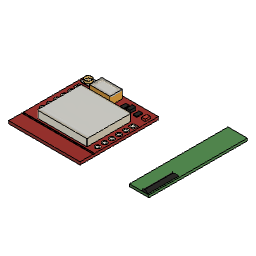
Sim800L Board + Antenna (Autodesk Fusion 360 design; units mm, degrees)
Autodesk Fusion 360 part; units mm, degrees
note: some values were not read from the file. Set by a fixed rule: which sketch regions a step uses.
sketch "Sketch1" plane through (0, 0, 0) normal (0, 0, 1) x (1, 0, 0)
  line L0 (12.75, 14) -> (-12.75, 14)
  line L1 (-12.75, 14) -> (-12.75, -14)
  line L2 (-12.75, -14) -> (12.75, -14)
  line L3 (12.75, -14) -> (12.75, 14)
  line L4 (12.75, 14) -> (-12.75, -14) construction
  line L5 (-12.75, 14) -> (12.75, -14) construction
  dimension "d1" = 25.5
  dimension "d2" = 28
  constraint horizontal L0
  constraint perpendicular L0 L1
  constraint parallel L0 L2
  constraint parallel L1 L3
  constraint coincident L4 origin
  constraint coincident L5 origin
  measures "d1" distance of L1.end L2.end
  measures "d2" distance of L0.end L1.end
extrude "Extrude1" add sketch "Sketch1" along normal blind 1 makes body 1
sketch "Sketch2" plane through (0, 0, 1) normal (0, 0, 1) x (-1, 0, 0)
  line L0 (-12.75, 14) -> (-12.75, -14)
  line L1 (-12.75, -14) -> (12.75, -14)
  line L2 (12.75, -14) -> (12.75, 14)
  line L3 (12.75, 14) -> (-12.75, 14)
  line L4 (12.75, 8.75) -> (-12.75, 8.75)
  line L5 (-12.75, 8.75) -> (-12.75, 9.25)
  line L6 (-12.75, 9.25) -> (12.75, 9.25)
  line L7 (12.75, 9.25) -> (12.75, 8.75)
  dimension "d5" = 0.5
  dimension "d6" = 4.75
  constraint horizontal L4
  constraint vertical L5
  constraint horizontal L6
  constraint vertical L7
  constraint coincident L0 L5.end
  constraint coincident L2 L4.start
  measures "d5" distance of L4.end L5.end
  measures "d6" distance of L3 L6
extrude "Extrude2" cut sketch "Sketch2" against normal blind 0.15 contours L0 L2 L4 L5 L6 L7 bodies 1
sketch "Sketch3" plane through (0, 0, 1) normal (0, 0, 1) x (-1, 0, 0)
  line L0 (12.75, 8.75) -> (-12.75, 8.75)
  line L1 (-12.75, 8.75) -> (-12.75, -14)
  line L2 (-12.75, -14) -> (12.75, -14)
  line L3 (12.75, -14) -> (12.75, 8.75)
  line L4 (8.45, -7.7) -> (-9.35, -7.7)
  line L5 (-9.35, -7.7) -> (-9.35, 8.1)
  line L6 (-9.35, 8.1) -> (8.45, 8.1)
  line L7 (8.45, 8.1) -> (8.45, -7.7)
  dimension "d9" = 17.8
  dimension "d10" = 15.8
  dimension "d11" = 3.4
  dimension "d12" = 6.8
  dimension "d13" = 6.3
  constraint horizontal L4
  constraint vertical L5
  constraint horizontal L6
  constraint vertical L7
  measures "d9" distance of L4.start L4.end
  measures "d10" distance of L4.end L5.end
  measures "d11" distance of L1 L5
  measures "d13" distance of L2 L4
extrude "Extrude3" add sketch "Sketch3" along normal blind 2.5 contours L4 L5 L6 L7 bodies 1
sketch "Sketch4" plane through (0, 0, 1) normal (0, 0, 1) x (-1, 0, 0)
  line L0 (8.45, 8.1) -> (8.45, -7.7)
  line L1 (8.45, -7.7) -> (-9.35, -7.7)
  line L2 (-9.35, -7.7) -> (-9.35, 8.1)
  line L3 (-9.35, 8.1) -> (8.45, 8.1)
  line L4 (12.75, 8.75) -> (-12.75, 8.75)
  line L5 (-12.75, 8.75) -> (-12.75, -14)
  line L6 (-12.75, -14) -> (12.75, -14)
  line L7 (12.75, -14) -> (12.75, 8.75)
  line L8 (6.45, -13) -> (-0.85, -13)
  line L9 (-0.85, -13) -> (-0.85, -8.6)
  line L10 (-0.85, -8.6) -> (6.45, -8.6)
  line L11 (6.45, -8.6) -> (6.45, -13)
  dimension "d16" = 4.4
  dimension "d17" = 7.3
  dimension "d18" = 1
  dimension "d19" = 6.3
  constraint horizontal L8
  constraint vertical L9
  constraint horizontal L10
  constraint vertical L11
  measures "d16" distance of L8.end L9.end
  measures "d17" distance of L8.start L8.end
  measures "d18" distance of L6 L8
  measures "d19" distance of L7 L11
extrude "Extrude4" add sketch "Sketch4" along normal blind 3 contours L8 L9 L10 L11 bodies 1
sketch "Sketch5" plane through (0, 0, 1) normal (0, 0, 1) x (-1, 0, 0)
  line L0 (6.45, -8.6) -> (6.45, -13)
  line L1 (6.45, -13) -> (-0.85, -13)
  line L2 (-0.85, -13) -> (-0.85, -8.6)
  line L3 (-0.85, -8.6) -> (6.45, -8.6)
  line L4 (8.45, 8.1) -> (8.45, -7.7)
  line L5 (8.45, -7.7) -> (-9.35, -7.7)
  line L6 (-9.35, -7.7) -> (-9.35, 8.1)
  line L7 (-9.35, 8.1) -> (8.45, 8.1)
  line L8 (12.75, 8.75) -> (-12.75, 8.75)
  line L9 (-12.75, 8.75) -> (-12.75, -14)
  line L10 (-12.75, -14) -> (12.75, -14)
  line L11 (12.75, -14) -> (12.75, 8.75)
  line L12 (-3.05, -12) -> (-4.35, -12)
  line L13 (-4.35, -12) -> (-4.35, -10)
  line L14 (-4.35, -10) -> (-3.05, -10)
  line L15 (-3.05, -10) -> (-3.05, -12)
  line L16 (-5.45, -12) -> (-6.75, -12)
  line L17 (-6.75, -12) -> (-6.75, -9.9)
  line L18 (-6.75, -9.9) -> (-5.45, -9.9)
  line L19 (-5.45, -9.9) -> (-5.45, -12)
  line L20 (-7.85, -12) -> (-9.15, -12)
  line L21 (-9.15, -12) -> (-9.15, -9.9)
  line L22 (-9.15, -9.9) -> (-7.85, -9.9)
  line L23 (-7.85, -9.9) -> (-7.85, -12)
  line L24 (-10.65, -11.9) -> (-11.95, -11.9)
  line L25 (-11.95, -11.9) -> (-11.95, -10.1)
  line L26 (-11.95, -10.1) -> (-10.65, -10.1)
  line L27 (-10.65, -10.1) -> (-10.65, -11.9)
  dimension "d22" = 2
  dimension "d23" = 1.3
  dimension "d24" = 2
  dimension "d25" = 9.7
  dimension "d26" = 1.3
  dimension "d27" = 2.1
  dimension "d28" = 7.3
  dimension "d29" = 2
  dimension "d30" = 2.1
  dimension "d31" = 1.3
  dimension "d32" = 2
  dimension "d33" = 4.9
  dimension "d34" = 1.3
  dimension "d35" = 1.8
  dimension "d36" = 2.1
  dimension "d37" = 2.1
  constraint horizontal L12
  constraint vertical L13
  constraint horizontal L14
  constraint vertical L15
  constraint horizontal L16
  constraint vertical L17
  constraint horizontal L18
  constraint vertical L19
  constraint horizontal L20
  constraint vertical L21
  constraint horizontal L22
  constraint vertical L23
  constraint horizontal L24
  constraint vertical L25
  constraint horizontal L26
  constraint vertical L27
  measures "d22" distance of L12.end L13.end
  measures "d23" distance of L12.start L12.end
  measures "d24" distance of L10 L12
  measures "d25" distance of L9 L15
  measures "d26" distance of L16.start L16.end
  measures "d27" distance of L16.end L17.end
  measures "d28" distance of L9 L19
  measures "d29" distance of L10 L16
  measures "d30" distance of L20.end L21.end
  measures "d31" distance of L20.start L20.end
  measures "d32" distance of L10 L20
  measures "d33" distance of L9 L23
  measures "d34" distance of L24.start L24.end
  measures "d35" distance of L24.end L25.end
  measures "d36" distance of L10 L24
  measures "d37" distance of L9 L27
extrude "Extrude5" add sketch "Sketch5" along normal blind 0.3 contours L12 L13 L14 L15 bodies 1
extrude "Extrude6" add sketch "Sketch5" along normal blind 1 contours L16 L17 L18 L19 bodies 1
extrude "Extrude7" add sketch "Sketch5" along normal blind 0.3 contours L20 L21 L22 L23 bodies 1
extrude "Extrude8" add sketch "Sketch5" along normal blind 0.75 contours L24 L25 L26 L27 bodies 1
sketch "Sketch6" plane through (0, 0, 1) normal (0, 0, 1) x (-1, 0, 0)
  circle A0 centre (10.58, -12.3) radius 1.25
  circle A1 centre (10.58, -12.3) radius 1.15
  circle A2 centre (10.58, -12.3) radius 0.25
  line L0 (12.08, -10.8) -> (9.08, -10.8)
  line L1 (9.08, -10.8) -> (9.08, -13.8)
  line L2 (9.08, -13.8) -> (12.08, -13.8)
  line L3 (12.08, -13.8) -> (12.08, -10.8)
  line L4 (12.08, -10.8) -> (9.08, -13.8) construction
  line L5 (9.08, -10.8) -> (12.08, -13.8) construction
  line L6 (-12.75, -14) -> (12.75, -14)
  line L7 (12.75, -14) -> (12.75, 8.75)
  point P0 (10.58, -12.3)
  dimension "d46" = 2.5
  dimension "d47" = 0.1
  dimension "d48" = 0.5
  dimension "d49" = 3
  dimension "d50" = 3
  dimension "d51" = 0.2
  dimension "d52" = 0.67
  constraint concentric A0 A1
  constraint concentric A0 A2
  constraint horizontal L0
  constraint perpendicular L0 L1
  constraint parallel L0 L2
  constraint parallel L1 L3
  constraint coincident L4 P0
  constraint coincident L5 P0
  constraint coincident P0 A0.centre
  measures "d46" diameter of A0
  measures "d47" distance of A0 A1
  measures "d48" diameter of A2
  measures "d49" distance of L0.start L0.end
  measures "d50" distance of L0.start L2.end
  measures "d51" distance of L2 L6
  measures "d52" distance of L3 L7
extrude "Extrude9" add sketch "Sketch6" along normal blind 1 contours A0 | A2 bodies 1
extrude "Extrude10" add sketch "Sketch6" along normal blind 0.2 bodies 1
sketch "Sketch7" plane through (0, 0, 1) normal (0, 0, 1) x (-1, 0, 0)
  line L0 (12.08, -13.8) -> (9.08, -13.8)
  line L1 (9.08, -13.8) -> (9.08, -10.8)
  line L2 (9.08, -10.8) -> (12.08, -10.8)
  line L3 (12.08, -10.8) -> (12.08, -13.8)
  line L4 (12.75, 8.75) -> (-12.75, 8.75)
  line L5 (-12.75, 8.75) -> (-12.75, -14)
  line L6 (-12.75, -14) -> (12.75, -14)
  line L7 (12.75, -14) -> (12.75, 8.75)
  line L8 (8.45, 8.1) -> (8.45, -7.7)
  line L9 (8.45, -7.7) -> (-9.35, -7.7)
  line L10 (-9.35, -7.7) -> (-9.35, 8.1)
  line L11 (-9.35, 8.1) -> (8.45, 8.1)
  line L12 (6.45, -8.6) -> (6.45, -13)
  line L13 (6.45, -13) -> (-0.85, -13)
  line L14 (-0.85, -13) -> (-0.85, -8.6)
  line L15 (-0.85, -8.6) -> (6.45, -8.6)
  line L16 (-3.05, -10) -> (-3.05, -12)
  line L17 (-3.05, -12) -> (-4.35, -12)
  line L18 (-4.35, -12) -> (-4.35, -10)
  line L19 (-4.35, -10) -> (-3.05, -10)
  line L20 (-5.45, -9.9) -> (-5.45, -12)
  line L21 (-5.45, -12) -> (-6.75, -12)
  line L22 (-6.75, -12) -> (-6.75, -9.9)
  line L23 (-6.75, -9.9) -> (-5.45, -9.9)
  line L24 (-7.85, -9.9) -> (-7.85, -12)
  line L25 (-7.85, -12) -> (-9.15, -12)
  line L26 (-9.15, -12) -> (-9.15, -9.9)
  line L27 (-9.15, -9.9) -> (-7.85, -9.9)
  line L28 (-10.65, -10.1) -> (-10.65, -11.9)
  line L29 (-10.65, -11.9) -> (-11.95, -11.9)
  line L30 (-11.95, -11.9) -> (-11.95, -10.1)
  line L31 (-11.95, -10.1) -> (-10.65, -10.1)
  line L32 (-11.25, 8.75) -> (-11.25, -14) construction
  line L33 (10.75, 8.75) -> (10.75, -14) construction
  circle A0 centre (-11.25, -6.5) radius 0.6
  circle A1 centre (-11.25, -3.96) radius 0.6
  circle A2 centre (-11.25, -1.42) radius 0.6
  circle A3 centre (-11.25, 1.12) radius 0.6
  circle A4 centre (-11.25, 3.66) radius 0.6
  circle A5 centre (-11.25, 6.2) radius 0.6
  circle A6 centre (10.75, -9) radius 0.6
  circle A7 centre (10.75, -6.46) radius 0.6
  circle A8 centre (10.75, -3.92) radius 0.6
  circle A9 centre (10.75, -1.38) radius 0.6
  circle A10 centre (10.75, 1.16) radius 0.6
  circle A11 centre (10.75, 3.7) radius 0.6
  dimension "d57" = 1.5
  dimension "d58" = 2
  dimension "d59" = 7.5
  dimension "d60" = 1.2
  dimension "d63" = -2.54
  dimension "d64" = 0
  dimension "d65" = 1.2
  dimension "d66" = 5
  dimension "d69" = 0
  dimension "d70" = 2.54
  constraint coincident L4 L32.start
  constraint coincident L6 L32.end
  constraint perpendicular L6 L32
  constraint coincident L4 L33.start
  constraint coincident L6 L33.end
  constraint perpendicular L6 L33
  constraint coincident L32 A0.centre
  constraint coincident L33 A6.centre
  measures "d57" distance of L5 L32
  measures "d58" distance of L7 L33
  measures "d59" distance of L32.end A0.centre
  measures "d60" diameter of A0
  measures "d65" diameter of A6
  measures "d66" distance of L6 A6.centre
extrude "Extrude11" cut sketch "Sketch7" against normal up to surface (1 mm away) contours A0 | A1 | A2 | A3 | A4 | A5 | A6 | A7 | A8 | A9 | A10 | A11 bodies 1
sketch "Sketch8" plane through (0, 0, 0) normal (0, 0, -1) x (1, 0, 0)
  circle A0 centre (11.25, -1.42) radius 0.6
  circle A1 centre (-10.75, 3.7) radius 0.6
  circle A2 centre (-10.75, -6.46) radius 0.6
  circle A3 centre (-10.75, -3.92) radius 0.6
  circle A4 centre (11.25, 6.2) radius 0.6
  circle A5 centre (11.25, -3.96) radius 0.6
  circle A6 centre (11.25, 1.12) radius 0.6
  circle A7 centre (-10.75, 1.16) radius 0.6
  circle A8 centre (-10.75, -9) radius 0.6
  circle A9 centre (-10.75, -1.38) radius 0.6
  circle A10 centre (11.25, 3.66) radius 0.6
  circle A11 centre (11.25, -6.5) radius 0.6
  line L0 (12.75, -14) -> (12.75, 14)
  line L1 (12.75, 14) -> (-12.75, 14)
  line L2 (-12.75, 14) -> (-12.75, -14)
  line L3 (-12.75, -14) -> (12.75, -14)
  line L4 (-7.35, -13.95) -> (8.05, -13.95)
  line L5 (8.05, -13.95) -> (8.05, 3.25)
  line L6 (8.05, 3.25) -> (3.25, 3.25)
  line L7 (3.25, 3.25) -> (3.25, 1.95)
  line L8 (3.25, 1.95) -> (-7.35, 1.95)
  line L9 (-7.35, 1.95) -> (-7.35, -13.95)
  dimension "d73" = 15.4
  dimension "d75" = 10.6
  dimension "d76" = 1.3
  dimension "d77" = 15.9
  dimension "d108" = 0.05
  dimension "d109" = 20.1
  constraint perpendicular L5 L6
  constraint perpendicular L6 L7
  constraint perpendicular L5 L8
  constraint horizontal L8
  constraint vertical L9
  measures "d73" distance of L4.start L4.end
  measures "d75" distance of L7.end L8.end
  measures "d76" distance of L6 L8
  measures "d77" distance of L4.start L8.end
  measures "d108" distance of L3 L4
  measures "d109" distance of L0.start L9
extrude "Extrude12" add sketch "Sketch8" along normal blind 1.3 contours L4 L5 L6 L7 L8 L9 bodies 1
ref_plane "WorkPlane1" through (0, 0, -0.4) normal (0, 0, -1) x (-1, 0, 0)
sketch "Sketch10" plane through (0, 0, -0.4) normal (0, 0, -1) x (1, 0, 0)
  line L0 (-6.85, -0.3) -> (5.15, -0.3)
  line L1 (5.15, -0.3) -> (5.15, -15.1)
  line L2 (5.15, -15.1) -> (-6.85, -15.1)
  line L3 (-6.85, -15.1) -> (-6.85, -0.3)
  line L4 (12.75, -14) -> (-12.75, -14)
  line L5 (-7.35, 1.95) -> (-7.35, -13.95)
  point P0 (-7.35, -13.95)
  dimension "d90" = 12
  dimension "d91" = 14.8
  dimension "d110" = 1.1
  dimension "d111" = 0.5
  constraint horizontal L0
  constraint vertical L1
  constraint horizontal L2
  constraint vertical L3
  measures "d90" distance of L0.start L0.end
  measures "d91" distance of L0.start L2.end
  measures "d110" distance of L1.end L4
  measures "d111" distance of L2.end L5
extrude "Extrude14" cut sketch "Sketch10" along normal blind 0.75 bodies 1
sketch "Sketch9" plane through (0, 0, -0.4) normal (0, 0, -1) x (1, 0, 0)
  line L0 (5.15, -0.25) -> (5.15, -12.25)
  line L1 (5.15, -12.25) -> (2.35, -15.05)
  line L2 (2.35, -15.05) -> (-6.85, -15.05)
  line L3 (-6.85, -15.05) -> (-6.85, -0.25)
  line L4 (-6.85, -0.25) -> (5.15, -0.25)
  line L5 (8.05, -13.95) -> (-7.35, -13.95)
  dimension "d82" = 12
  dimension "d83" = 9.2
  dimension "d84" = 45
  dimension "d96" = 14.8
  dimension "d112" = 1.1
  dimension "d113" = 0.5
  constraint perpendicular L0 L2
  constraint perpendicular L2 L3
  constraint perpendicular L0 L4
  measures "d82" distance of L0 L3
  measures "d83" distance of L1.end L2.end
  measures "d84" angle of L0 L1
  measures "d96" distance of L2.end L3.end
  measures "d112" distance of L2 L5
  measures "d113" distance of L3 L5.end
extrude "Extrude13" add sketch "Sketch9" along normal blind 0.7 separate body makes body 2
fillet "Fillet1" radius 0.5 5 edges at (2.35, 15.05, -0.75) (-6.85, 15.05, -0.75) (5.15, 12.25, -0.75) (5.15, 0.25, -0.75) (-6.85, 0.25, -0.75) on bodies 2
sketch "Sketch11" plane through (0, 0, 1) normal (0, 0, 1) x (-1, 0, 0)
  circle A0 centre (-11.25, -1.42) radius 0.6
  circle A1 centre (10.75, 3.7) radius 0.6
  circle A2 centre (10.75, -6.46) radius 0.6
  circle A3 centre (10.75, -3.92) radius 0.6
  circle A4 centre (-11.25, 6.2) radius 0.6
  circle A5 centre (-11.25, -3.96) radius 0.6
  circle A6 centre (-11.25, 1.12) radius 0.6
  circle A7 centre (10.75, 1.16) radius 0.6
  circle A8 centre (10.75, -9) radius 0.6
  circle A9 centre (10.75, -1.38) radius 0.6
  circle A10 centre (-11.25, 3.66) radius 0.6
  circle A11 centre (-11.25, -6.5) radius 0.6
  line L0 (12.08, -13.8) -> (9.08, -13.8)
  line L1 (9.08, -13.8) -> (9.08, -10.8)
  line L2 (9.08, -10.8) -> (12.08, -10.8)
  line L3 (12.08, -10.8) -> (12.08, -13.8)
  line L4 (12.75, 8.75) -> (-12.75, 8.75)
  line L5 (-12.75, 8.75) -> (-12.75, -14)
  line L6 (-12.75, -14) -> (12.75, -14)
  line L7 (12.75, -14) -> (12.75, 8.75)
  line L8 (8.45, 8.1) -> (8.45, -7.7)
  line L9 (8.45, -7.7) -> (-9.35, -7.7)
  line L10 (-9.35, -7.7) -> (-9.35, 8.1)
  line L11 (-9.35, 8.1) -> (8.45, 8.1)
  line L12 (6.45, -8.6) -> (6.45, -13)
  line L13 (6.45, -13) -> (-0.85, -13)
  line L14 (-0.85, -13) -> (-0.85, -8.6)
  line L15 (-0.85, -8.6) -> (6.45, -8.6)
  line L16 (-3.05, -10) -> (-3.05, -12)
  line L17 (-3.05, -12) -> (-4.35, -12)
  line L18 (-4.35, -12) -> (-4.35, -10)
  line L19 (-4.35, -10) -> (-3.05, -10)
  line L20 (-5.45, -9.9) -> (-5.45, -12)
  line L21 (-5.45, -12) -> (-6.75, -12)
  line L22 (-6.75, -12) -> (-6.75, -9.9)
  line L23 (-6.75, -9.9) -> (-5.45, -9.9)
  line L24 (-7.85, -9.9) -> (-7.85, -12)
  line L25 (-7.85, -12) -> (-9.15, -12)
  line L26 (-9.15, -12) -> (-9.15, -9.9)
  line L27 (-9.15, -9.9) -> (-7.85, -9.9)
  line L28 (-10.65, -10.1) -> (-10.65, -11.9)
  line L29 (-10.65, -11.9) -> (-11.95, -11.9)
  line L30 (-11.95, -11.9) -> (-11.95, -10.1)
  line L31 (-11.95, -10.1) -> (-10.65, -10.1)
  line L32 (-12.15, -7.4) -> (-10.35, -7.4)
  line L33 (-10.35, -7.4) -> (-10.35, -5.6)
  line L34 (-10.35, -5.6) -> (-12.15, -5.6)
  line L35 (-12.15, -5.6) -> (-12.15, -7.4)
  line L36 (-12.15, -7.4) -> (-10.35, -5.6) construction
  line L37 (-10.35, -7.4) -> (-12.15, -5.6) construction
  line L38 (9.85, -9.9) -> (11.65, -9.9)
  line L39 (11.65, -9.9) -> (11.65, -8.1)
  line L40 (11.65, -8.1) -> (9.85, -8.1)
  line L41 (9.85, -8.1) -> (9.85, -9.9)
  line L42 (9.85, -9.9) -> (11.65, -8.1) construction
  line L43 (11.65, -9.9) -> (9.85, -8.1) construction
  circle A12 centre (10.75, -6.46) radius 0.9
  circle A13 centre (10.75, -3.92) radius 0.9
  circle A14 centre (10.75, -1.38) radius 0.9
  circle A15 centre (10.75, 1.16) radius 0.9
  circle A16 centre (10.75, 3.7) radius 0.9
  circle A17 centre (-11.25, 6.2) radius 0.9
  circle A18 centre (-11.25, 3.66) radius 0.9
  circle A19 centre (-11.25, 1.12) radius 0.9
  circle A20 centre (-11.25, -1.42) radius 0.9
  circle A21 centre (-11.25, -3.96) radius 0.9
  point P0 (-11.25, -6.5)
  point P1 (10.75, -9)
  dimension "d97" = 1.8
  dimension "d98" = 1.8
  dimension "d99" = 1.8
  dimension "d100" = 1.8
  dimension "d103" = 1.8
  dimension "d104" = 1.8
  constraint horizontal L32
  constraint perpendicular L32 L33
  constraint parallel L32 L34
  constraint parallel L33 L35
  constraint coincident L36 P0
  constraint coincident L37 P0
  constraint coincident P0 A11.centre
  constraint horizontal L38
  constraint perpendicular L38 L39
  constraint parallel L38 L40
  constraint parallel L39 L41
  constraint coincident L42 P1
  constraint coincident L43 P1
  constraint coincident P1 A8.centre
  constraint concentric A2 A12
  constraint concentric A3 A13
  constraint concentric A9 A14
  constraint concentric A7 A15
  constraint concentric A1 A16
  constraint concentric A4 A17
  constraint concentric A10 A18
  constraint concentric A6 A19
  constraint concentric A0 A20
  constraint concentric A5 A21
  constraint equal A12 A14
  constraint equal A14 A15
  constraint equal A15 A16
  constraint equal A16 A21
  constraint equal A20 A21
  constraint equal A19 A20
  constraint equal A18 A19
  constraint equal A17 A18
  measures "d97" distance of L33.end L34.end
  measures "d98" distance of L32.end L33.end
  measures "d99" distance of L39.end L40.end
  measures "d100" distance of L38.end L39.end
  measures "d103" diameter of A12
  measures "d104" diameter of A13
extrude "Extrude15" cut sketch "Sketch11" against normal blind 0.01 contours L32 L33 L34 L35 | L38 L39 L40 L41 | A12 | A13 | A14 | A15 | A16 | A17 | A18 | A19 | A20 | A21 bodies 1
fillet "Fillet2" radius 0.2 4 edges at (-12.08, 13.8, 1.1) (-9.08, 13.8, 1.1) (-12.08, 10.8, 1.1) (-9.08, 10.8, 1.1) on bodies 1
fillet "Fillet3" radius 0.3 4 edges at (9.35, -8.1, 2.25) (-8.45, -8.1, 2.25) (9.35, 7.7, 2.25) (-8.45, 7.7, 2.25) on bodies 1
sketch "Sketch12" plane through (0, 0, 0) normal (0, 0, 1) x (1, 0, 0)
  line L0 (28.2729, 23.3773) -> (35.1729, 23.3773)
  line L1 (35.1729, 23.3773) -> (35.1729, -11.8227)
  line L2 (35.1729, -11.8227) -> (28.2729, -11.8227)
  line L3 (28.2729, -11.8227) -> (28.2729, 23.3773)
  dimension "d114" = 35.2
  dimension "d115" = 6.9
  constraint horizontal L0
  constraint vertical L1
  constraint horizontal L2
  constraint vertical L3
  measures "d114" distance of L0.end L1.end
  measures "d115" distance of L0.start L0.end
extrude "Extrude16" add sketch "Sketch12" along normal blind 0.85 separate body makes body 3
sketch "Sketch13" plane through (0, 0, 0.85) normal (0, 0, 1) x (-1, 0, 0)
  line L0 (-28.2729, 11.8227) -> (-35.1729, 11.8227)
  line L1 (-35.1729, 11.8227) -> (-35.1729, -23.3773)
  line L2 (-35.1729, -23.3773) -> (-28.2729, -23.3773)
  line L3 (-28.2729, -23.3773) -> (-28.2729, 11.8227)
  line L4 (-32.6729, 0.8227) -> (-34.6729, 0.8227)
  line L5 (-34.6729, 0.8227) -> (-34.6729, 11.8127)
  line L6 (-34.6729, 11.8127) -> (-32.6729, 11.8127)
  line L7 (-32.6729, 11.8127) -> (-32.6729, 0.8227)
  dimension "d118" = 2
  dimension "d119" = 0.5
  dimension "d120" = 11
  dimension "d124" = 0.01
  constraint horizontal L4
  constraint vertical L5
  constraint horizontal L6
  constraint vertical L7
  measures "d118" distance of L4.start L4.end
  measures "d119" distance of L1 L5.end
  measures "d120" distance of L0 L4.end
  measures "d124" distance of L0 L6
extrude "Extrude17" add sketch "Sketch13" along normal blind 1 contours L4 L5 L6 L7 bodies 3
fillet "Fillet4" radius 0.99 3 edges at (32.6729, -6.3177, 1.85) (34.6729, -6.3177, 1.85) (33.6729, -0.8227, 1.85) on bodies 3
sketch "Sketch14" plane through (0, 0, 0) normal (0, 0, -1) x (1, 0, 0)
  line L0 (-7.35, 1.95) -> (3.25, 1.95)
  line L1 (3.25, 1.95) -> (3.25, 3.25)
  line L2 (3.25, 3.25) -> (8.05, 3.25)
  line L3 (8.05, 3.25) -> (8.05, -13.95)
  line L4 (8.05, -13.95) -> (-7.35, -13.95)
  line L5 (-7.35, -13.95) -> (-7.35, 1.95)
  circle A0 centre (11.25, -1.42) radius 0.6
  circle A1 centre (-10.75, 3.7) radius 0.6
  circle A2 centre (-10.75, -6.46) radius 0.6
  circle A3 centre (-10.75, -3.92) radius 0.6
  circle A4 centre (11.25, 6.2) radius 0.6
  circle A5 centre (11.25, -3.96) radius 0.6
  circle A6 centre (11.25, 1.12) radius 0.6
  circle A7 centre (-10.75, 1.16) radius 0.6
  circle A8 centre (-10.75, -9) radius 0.6
  circle A9 centre (-10.75, -1.38) radius 0.6
  circle A10 centre (11.25, 3.66) radius 0.6
  circle A11 centre (11.25, -6.5) radius 0.6
  line L6 (12.75, -14) -> (12.75, 14)
  line L7 (12.75, 14) -> (-12.75, 14)
  line L8 (-12.75, 14) -> (-12.75, -14)
  line L9 (-12.75, -14) -> (12.75, -14)
  circle A12 centre (-10.75, 3.7) radius 0.9
  circle A13 centre (-10.75, 1.16) radius 0.9
  circle A14 centre (-10.75, -1.38) radius 0.9
  circle A15 centre (-10.75, -3.92) radius 0.9
  circle A16 centre (-10.75, -6.46) radius 0.9
  circle A17 centre (-10.75, -9) radius 0.9
  circle A18 centre (11.25, -6.5) radius 0.9
  circle A19 centre (11.25, -3.96) radius 0.9
  circle A20 centre (11.25, -1.42) radius 0.9
  circle A21 centre (11.25, 1.12) radius 0.9
  circle A22 centre (11.25, 3.66) radius 0.9
  circle A23 centre (11.25, 6.2) radius 0.9
  dimension "d125" = 1.8
  constraint concentric A1 A12
  constraint concentric A7 A13
  constraint concentric A9 A14
  constraint concentric A3 A15
  constraint concentric A2 A16
  constraint concentric A8 A17
  constraint concentric A11 A18
  constraint concentric A5 A19
  constraint concentric A0 A20
  constraint concentric A6 A21
  constraint concentric A10 A22
  constraint concentric A4 A23
  constraint equal A12 A13
  constraint equal A13 A14
  constraint equal A14 A15
  constraint equal A15 A16
  constraint equal A16 A17
  constraint equal A17 A18
  constraint equal A18 A19
  constraint equal A19 A20
  constraint equal A20 A21
  constraint equal A21 A22
  constraint equal A22 A23
  measures "d125" diameter of A12
extrude "Extrude18" cut sketch "Sketch14" against normal blind 0.01 contours A12 | A13 | A14 | A15 | A16 | A17 | A18 | A19 | A20 | A21 | A22 | A23 bodies 1
named bodies: "PCB", "SIM", "Antenna"
